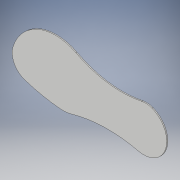
# Autodesk Inventor part: lateral
Saved by Autodesk Inventor 2019 (Build 230136000, 136)
## iProperties
Created: 2020-02-14
Part Number: lateral
Material: Genérico
Document SubType Name: Modeling
Designer: Mafer1
Density: 1 g/cm^3
Appearance: Valor por defecto
Author: Mafer1
Autodesk Inventor part; units mm, degrees
ref_plane "YZ Plane" through (0, 0, 0) normal (1, 0, 0) x (0, 1, 0)
ref_plane "XZ Plane" through (0, 0, 0) normal (0, 1, 0) x (-1, 0, 0)
ref_plane "XY Plane" through (0, 0, 0) normal (0, 0, 1) x (1, 0, 0)
sketch "Boceto1" plane through (0, 0, 0) normal (0, 0, 1) x (1, 0, 0)
  circle A0 centre (0, 0) radius 55
  circle A1 centre (-250, 0) radius 90
  circle A2 centre (-350, -15) radius 55
  arc A3 (-367.327, -67.1994) -> (-257.5001, -89.6869) centre (-217.9996, 382.6643) ccw
  arc A4 (-67.4485, -46.375) -> (19.7456, 51.3333) centre (-5.3852, -14) ccw
  arc A5 (-21.7116, -82.0694) -> (-225.2051, -86.5171) centre (-115.0054, -471.0376) ccw
  arc A6 (-203.0142, 76.7616) -> (-402.5986, 1.0743) centre (-273.4929, -38.3808) ccw
  arc A7 (-211.1659, 81.3704) -> (-11.2574, 53.8356) centre (-72.6616, 347.4842) ccw
  dimension "d0" = 110
  dimension "d1" = 180
  dimension "d2" = 250
  dimension "d11" = 110
  dimension "d12" = 100
  dimension "d13" = 15
  dimension "d16" = 474
  dimension "d17" = 70
  dimension "d20" = 14
  dimension "d21" = 400
  dimension "d22" = 135
  dimension "d23" = 300
  dimension "d24" = 46.375
  constraints: 19 point on circle, 9 tangent, 8 centre point, 1 coincident, 1 horizontal alignment
  measures "d0" diameter of A0
  measures "d1" diameter of A1
  measures "d2" distance of point (0, 0) A1.centre
  measures "d11" diameter of A2
  measures "d12" horizontal distance of A1.centre A2.centre
  measures "d13" vertical distance of A2.centre A1.centre
  measures "d16" radius of A3
  measures "d17" radius of A4
  measures "d20" vertical distance of A4.centre point (0, 0)
  measures "d21" radius of A5
  measures "d22" radius of A6
  measures "d23" radius of A7
  measures "d24" vertical distance of A4.start point (0, 0)
extrude "Extrusión1" add sketch "Boceto1" along normal blind 3.3
equation "\"d11\" = d0"
